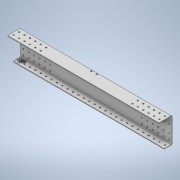
# Autodesk Inventor part: front-back pannel 00000
Saved by Autodesk Inventor 2022 (Build 260153000, 153)
## iProperties
Created: 2022-01-13
Part Number: front-back pannel 00000
Material: Generic
Document SubType Name: Sheet Metal
Designer: Jacob
Density: 1 g/cm^3
Sheet Metal Rule: Default
Appearance: Default
Sheet Metal Width: 8.315 in
Sheet Metal Length: 28.000 in
Sheet Metal Area: 232.834 in^2
Flat Pattern Width: 21.1213 cm
Flat Pattern Length: 71.12 cm
Flat Pattern Area: 1502.15 cm^2
Author: Jacob
Autodesk Inventor part; units mm, degrees
ref_plane "YZ Plane" through (0, 0, 0) normal (1, 0, 0) x (0, 1, 0)
ref_plane "XZ Plane" through (0, 0, 0) normal (0, 1, 0) x (-1, 0, 0)
ref_plane "XY Plane" through (0, 0, 0) normal (0, 0, 1) x (1, 0, 0)
sketch "Sketch1" plane through (0, 0, 0) normal (0, 0, 1) x (1, 0, 0)
  line L0 (0, 0) -> (711.2, 0)
  line L1 (711.2, 0) -> (711.2, 120.65)
  line L2 (711.2, 120.65) -> (0, 120.65)
  line L3 (0, 120.65) -> (0, 0)
  dimension "d0" = 711.2
  dimension "d1" = 120.65
  measures "d0" distance of L2.end L1.end
  measures "d1" distance of L1.end L0.end
extrude "Plate1" add sketch "Sketch1" along normal blind 3.175
sketch "Sketch2" plane through (0, 117.475, 0) normal (0, 1, 0) x (-1, 0, 0)
  line L0 (-711.2, 0) -> (0, 0)
  line L1 (0, 0) -> (0, 63.5)
  line L2 (0, 63.5) -> (-711.2, 63.5)
  line L3 (-711.2, 63.5) -> (-711.2, 0)
  constraints: 6 end point, 1 horizontal, 1 perpendicular, 1 vertical
edge flange "Flange1" height 63.5 angle 90 thickness 3.175 bend radius 3.175 thickness toward (0, 1, 0) relief tear relief width 3.175 relief depth 1.5875 edges at (355.6, 120.65, 3.175) wall of the first edge with corners at (711.2, 117.475, 0) (0, 117.475, 0) (0, 117.475, 63.5) (711.2, 117.475, 63.5)
bend "Bend1"
corner "Corner1"
sketch "Sketch3" plane through (711.2, 3.175, 0) normal (0, -1, 0) x (1, 0, 0)
  line L0 (-711.2, 0) -> (0, 0)
  line L1 (0, 0) -> (0, 38.1)
  line L2 (0, 38.1) -> (-711.2, 38.1)
  line L3 (-711.2, 38.1) -> (-711.2, 0)
  constraints: 6 end point, 1 horizontal, 1 perpendicular, 1 vertical
edge flange "Flange2" height 38.1 angle 90 thickness 3.175 bend radius 3.175 thickness toward (0, -1, 0) relief tear relief width 3.175 relief depth 1.5875 edges at (355.6, 0, 3.175) wall of the first edge with corners at (0, 3.175, 0) (711.2, 3.175, 0) (711.2, 3.175, 38.1) (0, 3.175, 38.1)
bend "Bend2"
corner "Corner2"
sketch "Sketch5" plane through (0, 0, 38.1) normal (0, -1, 0) x (1, 0, 0)
  line L0 (0, -31.75) -> (0, 0) projected
  circle A0 centre (12.7, -15.748) radius 3.302
  line L1 (711.2, -38.1) -> (0, -38.1) projected
  dimension "d129" = 6.604
  dimension "d237" = 12.7
  dimension "d238" = 22.352
  constraints: 1 centre point
  measures "d129" diameter of A0
  measures "d237" distance from line of L0 A0.centre
  measures "d238" distance from line of L1 A0.centre
sketch "Sketch11" plane through (0, 0, 0) normal (0, 0, -1) x (-1, 0, 0)
  circle A0 centre (-12.7, 104.775) radius 3.302
  line L0 (0, 114.3) -> (0, 6.35) projected
  circle A1 centre (-12.7, 15.875) radius 3.302
  line L1 (0, 0) -> (-711.2, 0) projected
  circle A2 centre (-12.7, 41.275) radius 3.302
  circle A3 centre (-12.7, 79.375) radius 3.302
  circle A4 centre (-698.5, 15.875) radius 3.302
  line L2 (-711.2, 6.35) -> (-711.2, 114.3) projected
  circle A5 centre (-698.5, 41.275) radius 3.302
  circle A6 centre (-698.5, 79.375) radius 3.302
  circle A7 centre (-698.5, 104.775) radius 3.302
  dimension "d177" = 6.604
  dimension "d178" = 12.7
  dimension "d179" = 6.604
  dimension "d180" = 12.7
  dimension "d181" = 15.875
  dimension "d182" = 6.604
  dimension "d183" = 25.4
  dimension "d184" = 6.604
  dimension "d185" = 38.1
  dimension "d186" = 25.4
  dimension "d187" = 6.604
  dimension "d188" = 15.875
  dimension "d189" = 12.7
  dimension "d190" = 6.604
  dimension "d191" = 6.604
  dimension "d192" = 6.604
  dimension "d193" = 25.4
  dimension "d194" = 38.1
  dimension "d195" = 25.4
  constraints: 8 centre point
  measures "d177" diameter of A0
  measures "d178" distance from line of L0 A0.centre
  measures "d179" diameter of A1
  measures "d180" distance from line of L0 A1.centre
  measures "d181" distance from line of L1 A1.centre
  measures "d182" diameter of A2
  measures "d183" distance of A1.centre A2.centre
  measures "d184" diameter of A3
  measures "d185" distance of A2.centre A3.centre
  measures "d186" distance of A0.centre A3.centre
  measures "d187" diameter of A4
  measures "d188" distance from line of L1 A4.centre
  measures "d189" distance from line of L2 A4.centre
  measures "d190" diameter of A5
  measures "d191" diameter of A6
  measures "d192" diameter of A7
  measures "d193" distance of A4.centre A5.centre
  measures "d194" distance of A6.centre A5.centre
  measures "d195" distance of A7.centre A6.centre
extrude "Cut11" cut sketch "Sketch11" against normal blind 3.175
pattern_linear "Rectangular Pattern11" count 6 spacing 25.4 along (1, 0, 0) count 6 spacing 25.4 along (-1, 0, 0) of "Cut11"
sketch "Sketch12" plane through (0, 120.65, 63.5) normal (0, 1, 0) x (1, 0, 0)
  circle A0 centre (12.7, 15.748) radius 3.302
  line L0 (711.2, 0) -> (0, 0) projected
  line L1 (0, 0) -> (0, 57.15) projected
  circle A1 centre (12.7, 41.148) radius 3.302
  circle A2 centre (698.5, 15.748) radius 3.302
  line L2 (711.2, 57.15) -> (711.2, 0) projected
  circle A3 centre (698.5, 41.148) radius 3.302
  point P0 (0, 63.5)
  dimension "d204" = 6.604
  dimension "d205" = 15.748
  dimension "d206" = 12.7
  dimension "d207" = 6.604
  dimension "d208" = 25.4
  dimension "d209" = 12.7
  dimension "d210" = 6.604
  dimension "d211" = 15.748
  dimension "d212" = 12.7
  dimension "d213" = 6.604
  dimension "d214" = 25.4
  dimension "d215" = 12.7
  constraints: 4 centre point
  measures "d204" diameter of A0
  measures "d205" distance from line of L0 A0.centre
  measures "d206" distance from line of L1 A0.centre
  measures "d207" diameter of A1
  measures "d208" distance of A0.centre A1.centre
  measures "d209" distance from line of L1 A1.centre
  measures "d210" diameter of A2
  measures "d211" distance from line of L0 A2.centre
  measures "d212" distance from line of L2 A2.centre
  measures "d213" diameter of A3
  measures "d214" distance of A2.centre A3.centre
  measures "d215" distance from line of L2 A3.centre
extrude "Cut12" cut sketch "Sketch12" against normal blind 3.175
pattern_linear "Rectangular Pattern12" count 6 spacing 25.4 along (-1, 0, 0) count 6 spacing 25.4 along (1, 0, 0) of "Cut12"
sketch "Sketch13" plane through (0, 120.65, 63.5) normal (0, 1, 0) x (1, 0, 0)
  line L0 (711.2, 0) -> (0, 0) projected
  line L1 (355.6, 0) -> (355.6, 109.3698)
  circle A0 centre (342.9, 50.8) radius 3.302
  line L2 (0, 63.5) -> (711.2, 63.5) projected
  circle A1 centre (368.3, 50.8) radius 3.302
  dimension "d224" = 6.604
  dimension "d225" = 12.7
  dimension "d226" = 12.7
  dimension "d227" = 6.604
  dimension "d228" = 12.7
  dimension "d229" = 12.7
  constraints: 2 centre point, 2 end point, 1 midpoint, 1 vertical
  measures "d224" diameter of A0
  measures "d225" distance from line of L1 A0.centre
  measures "d226" distance from line of L2 A0.centre
  measures "d227" diameter of A1
  measures "d228" distance from line of L1 A1.centre
  measures "d229" distance from line of L2 A1.centre
extrude "Cut13" cut sketch "Sketch13" against normal blind 3.175
extrude "Cut14" cut sketch "Sketch5" against normal blind 3.175
pattern_linear "Rectangular Pattern14" count 28 spacing 25.4 along (1, 0, 0) of "Cut14"
equation "\"d196\" = Thickness"
equation "\"d216\" = Thickness"
equation "\"d230\" = Thickness"
equation "\"d232\" = Thickness"
equation "\"d2\" = Thickness"
equation "\"d3\" = BendReliefWidth"
equation "\"d4\" = BendReliefDepth"
equation "\"d5\" = MinimumRemnant"
equation "\"d6\" = TransitionRadius"
equation "\"d9\" = BendRadius"
equation "\"d10\" = CornerReliefSize"
equation "\"d11\" = GapSize"
equation "\"d12\" = JacobiRadiusSize"
equation "\"d13\" = BendReliefWidth"
equation "\"d14\" = BendReliefDepth"
equation "\"d15\" = MinimumRemnant"
equation "\"d16\" = TransitionRadius"
equation "\"d19\" = BendRadius"
equation "\"d20\" = CornerReliefSize"
equation "\"d21\" = GapSize"
equation "\"d22\" = JacobiRadiusSize"
equation "\"BendRadius\" = Thickness"
equation "\"BendReliefWidth\" = Thickness"
equation "\"BendReliefDepth\" = 0.5 * Thickness"
equation "\"CornerReliefSize\" = 4 * Thickness"
equation "\"MinimumRemnant\" = 2 * Thickness"
equation "\"TransitionRadius\" = BendRadius"
equation "\"JacobiRadiusSize\" = BendRadius"
equation "\"GapSize\" = Thickness"
equation "\"Thickness\" = 3.175"
body "Solid1"
